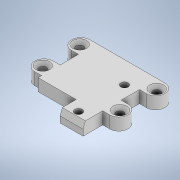
# Autodesk Inventor part: Крепление мотора
Saved by Autodesk Inventor 2020 (Build 240168000, 168)
## iProperties
Created: 2021-05-23
Part Number: Крепление мотора
Material: Типовые
Document SubType Name: Modeling
Designer: Антон
Density: 1 g/cm^3
Appearance: По умолчанию
Author: Антон
Autodesk Inventor part; units mm, degrees
ref_plane "YZ Plane" through (0, 0, 0) normal (1, 0, 0) x (0, 1, 0)
ref_plane "XZ Plane" through (0, 0, 0) normal (0, 1, 0) x (-1, 0, 0)
ref_plane "XY Plane" through (0, 0, 0) normal (0, 0, 1) x (1, 0, 0)
sketch "Эскиз1" plane through (0, 0, 0) normal (0, 1, 0) x (-1, 0, 0)
  line L0 (0, 0) -> (26.5, 0)
  line L1 (26.5, 0) -> (26.5, -32.524)
  line L2 (26.5, -32.524) -> (0, -32.524)
  line L3 (0, -32.524) -> (0, 0)
  dimension "d0" = 26.5
  dimension "d1" = 32.524
  constraints: 8 end point, 2 parallel, 1 horizontal, 1 perpendicular
  measures "d0" distance of L1.end L2.end
  measures "d1" distance of L0.end L1.end
extrude "Выдавливание1" add sketch "Эскиз1" along normal blind 5.3
sketch "Эскиз2" plane through (0, 5.3, 0) normal (0, 1, 0) x (1, 0, 0)
  line L0 (0, 13) -> (-5, 13)
  line L1 (-5, 13) -> (-5, 3)
  line L2 (-5, 13) -> (-5, 23)
  line L3 (-26.5, 32.524) -> (-26.5, 0) projected
  line L4 (0, 0) -> (0, 32.524) projected
  line L5 (-26.5, 0) -> (0, 0) projected
  dimension "d4" = 5
  dimension "d5" = 10
  dimension "d28" = 13
  constraints: 6 end point, 2 vertical, 1 collinear, 1 horizontal
  measures "d4" distance of L0.start L0.end
  measures "d5" distance of L0.end L1.end
  measures "d28" distance between parallel lines of L5 L0
hole "Отверстие1" at (-5, 5.3, -3) at (-5, 5.3, -23) direction (0, -1, 0) diameter 3.2 end through all
sketch "Эскиз3" plane through (0, 0, 0) normal (0, -1, 0) x (1, 0, 0)
  line L0 (-26.5, 0) -> (0, 0) projected
  line L1 (0, -8.524) -> (7, -8.524)
  line L2 (7, -8.524) -> (7, -16.524)
  line L3 (7, -16.524) -> (0, -16.524)
  line L4 (0, -16.524) -> (0, -8.524)
  line L5 (0, -32.524) -> (-26.5, -32.524) projected
  line L6 (0, 0) -> (0, -32.524) projected
  line L7 (0, 0) -> (0, -32.524) projected
  dimension "d13" = 7
  dimension "d14" = 8
  dimension "d27" = 16
  constraints: 8 end point, 2 parallel, 1 collinear, 1 horizontal, 1 perpendicular
  measures "d13" distance of L2.end L3.end
  measures "d14" distance of L1.end L2.end
  measures "d27" distance between parallel lines of L5 L3
extrude "Выдавливание2" add sketch "Эскиз3" against normal blind 5.3
sketch "Эскиз4" plane through (0, 5.3, 0) normal (0, 1, 0) x (1, 0, 0)
  line L0 (-26.5, 0) -> (0, 0) projected
  line L1 (7, 16.524) -> (7, 8.524) projected
  line L2 (7, 12.524) -> (0, 12.524)
  line L3 (0, 16.524) -> (0, 32.524) projected
  point P0 (3.5, 12.524)
  constraints: 2 end point, 2 midpoint, 1 horizontal, 1 point on line
hole "Отверстие2" at (3.5, 5.3, -12.524) direction (0, -1, 0) diameter 3.2 end through all countersink diameter 6 countersink angle 90
fillet "Сопряжение1" radius 4 2 edges at (7, 2.65, -16.524) (7, 2.65, -8.524)
ref_plane "РабПлоскость1" through (0, 0, -20.524) normal (0, 0, 1) x (1, 0, 0)
mirror "Зеркальное отражение1" about plane through (0, 0, -20.524) normal (0, 0, 1) of "Сопряжение1", "Отверстие2", "Выдавливание2"
ref_plane "РабПлоскость2" through (-13.25, 0, -16.524) normal (1, 0, 0) x (0, 0, -1)
mirror "Зеркальное отражение2" about plane through (-13.25, 0, -16.524) normal (1, 0, 0) of "Отверстие2", "Сопряжение1", "Выдавливание2", "Зеркальное отражение1"
sketch "Эскиз5" plane through (0, 5.3, 0) normal (0, 1, 0) x (1, 0, 0)
  line L0 (-26.5, 0) -> (0, 0) projected
  line L1 (-26.5, 0) -> (-10, 0)
  line L2 (-10, 0) -> (-10, 7)
  line L3 (-10, 7) -> (-26.5, 7)
  line L4 (-26.5, 7) -> (-26.5, 0)
  point P0 (-10, 0)
  dimension "d29" = 7
  dimension "d30" = 16.5
  constraints: 8 end point, 2 parallel, 1 horizontal, 1 perpendicular
  measures "d29" distance of L2.end L1.end
  measures "d30" distance of L2.end L3.end
extrude "Выдавливание3" cut sketch "Эскиз5" against normal through all
chamfer "Фаска1" distance 1 distance2 2.65 1 edges at (-5, 5.3, 0) measured on face at (-5, 5.3, -0.5)
